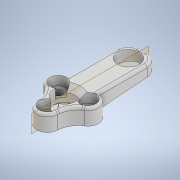
# Autodesk Inventor part: motorholder2
Saved by Autodesk Inventor 2020 (Build 240168000, 168)
## iProperties
Created: 2020-03-28
Part Number: motorholder2
Material: Generic
Document SubType Name: Modeling
Designer: Adam
Density: 1 g/cm^3
Appearance: Default
Author: Adam
Autodesk Inventor part; units mm, degrees
ref_plane "XZ Plane" through (0, 0, 0) normal (0, 1, 0) x (-1, 0, 0)
ref_plane "XY Plane" through (0, 0, 0) normal (0, 0, 1) x (1, 0, 0)
sketch "Sketch2" plane through (0, 0, 0) normal (0, 1, 0) x (-1, 0, 0)
  line L0 (0, 0) -> (10, 0)
  line L1 (10, 0) -> (10, -20)
  line L2 (10, -20) -> (0, -20)
  line L3 (0, -20) -> (0, 0)
  dimension "d0" = 20
  dimension "d1" = 10
  constraints: 8 end point, 2 parallel, 1 horizontal, 1 perpendicular
  measures "d0" distance of L0.end L1.end
  measures "d1" distance of L1.end L2.end
extrude "Extrusion1" add sketch "Sketch2" along normal blind 3
sketch "Sketch3" plane through (0, 3, 0) normal (0, 1, 0) x (1, 0, 0)
  line L0 (-10, 20) -> (-10, 0) projected
  line L1 (0, 20) -> (-10, 20) projected
  line L2 (-10, 0) -> (0, 0) projected
  circle A0 centre (-5, 2.25) radius 0.8
  circle A1 centre (-5, 2.25) radius 1.5
  circle A2 centre (-5, 5.43) radius 2
  point P0 (-4.278066, 3.564843)
  point P1 (-5.721934, 3.564843)
  dimension "d4" = 5
  dimension "d7" = 0
  dimension "d8" = 3.18
  dimension "d10" = 1.6
  dimension "d11" = 2.25
  dimension "d12" = 3
  dimension "d13" = 4
  constraints: 3 centre point, 3 coincident
  measures "d4" distance from line of L0 point (-5, 5.43)
  measures "d7" horizontal distance of point (-5, 5.43) point (-5, 2.25)
  measures "d8" distance of point (-5, 5.43) point (-5, 2.25)
  measures "d10" diameter of A0
  measures "d11" distance from line of L2 A0.centre
  measures "d12" diameter of A1
  measures "d13" diameter of A2
extrude "Extrusion2" cut sketch "Sketch3" against normal through all contours A0
pattern_circular "Circular Pattern1" count 3 over 360 about axis through (-5, 3, -5.43) along (0, 1, 0) of "Extrusion2"
ref_plane "Work Plane2" through (0, 1.3, 0) normal (0, -1, 0) x (1, 0, 0)
ref_plane "Work Plane1" through (0, 0, 0) normal (0, -1, 0) x (1, 0, 0)
extrude "Extrusion3" cut sketch "Sketch3" against normal up to surface (1.7 mm away) contours A0 | A1 A2 | A2 A1 picked at (-5.473989, 3.306122) picked at (-4.949872, 3.544237)
extrude "Extrusion4" cut sketch "Sketch3" against normal through all contours A2 A1 | A1 A2 picked at (-4.949872, 3.544237) picked at (-4.946615, 6.191119)
pattern_circular "Circular Pattern2" count 3 over 360 about axis through (-5, 3, -5.43) along (0, 1, 0) of "Extrusion4", "Extrusion3"
sketch "Sketch6" plane through (0, 3, 0) normal (0, 1, 0) x (1, 0, 0)
  arc A0 (-6.254307, 6.987792) -> (-6.97624, 5.737366) centre (-7.753961, 7.02) ccw
  circle A1 centre (-7.753961, 7.02) radius 1.925
  arc A2 (-3.745693, 6.987792) -> (-6.254307, 6.987792) centre (-5, 5.43) ccw
  circle A3 centre (-5, 2.25) radius 1.925
  circle A4 centre (-2.246039, 7.02) radius 1.925
  arc A5 (-6.923446, 2.172663) -> (-8.78266, 5.392916) centre (-10.920216, 2.011961) ccw
  arc A6 (-1.21734, 5.392916) -> (-3.076554, 2.172663) centre (0.920216, 2.011961) ccw
  arc A7 (-6.859214, 8.724422) -> (-3.140786, 8.724422) centre (-5, 12.266077) ccw
  line L0 (-7.753961, 8.945) -> (-7.753961, 22.712263)
  line L1 (-7.753961, 22.712263) -> (-16.279981, 22.712263)
  line L2 (-16.279981, 22.712263) -> (-16.279981, -9.843768)
  line L3 (-16.279981, -9.843768) -> (12.206544, -9.843768)
  line L4 (12.206544, -9.843768) -> (12.206544, 22.712263)
  line L5 (12.206544, 22.712263) -> (-2.592848, 22.712263)
  line L6 (-2.246039, 8.945) -> (-2.246039, 22.712263)
  point P0 (0, 0)
  point P1 (-1.21734, 5.392916)
  point P2 (-3.076554, 2.172663)
  dimension "d35" = 0.425
  dimension "d38" = 360
  dimension "d40" = 4
  dimension "d43" = 360
  constraints: 14 end point, 8 point on circle, 4 centre point, 4 perpendicular, 3 point on line, 2 vertical, 1 coincident, 1 tangent, 27 other
  measures "d35" radial gap between concentric circles of A1 A0
  measures "d40" radius of A5
extrude "Extrusion5" cut sketch "Sketch6" against normal through all contours A1 A5 A3 A6 A4 L6 L5 L4 L3 L2 L1 L0
fillet "Fillet1" radius 0.5 5 edges at (-5, 3, -0.325) (-2.5439, 3, -4.012) (-0.397, 3, -7.5555) (-9.603, 3, -7.5555) (-7.4561, 3, -4.012)
sketch "Sketch7" plane through (0, 3, 0) normal (0, 1, 0) x (1, 0, 0)
  point P0 (0, 0)
  point P1 (-5.030866, 17.338478)
hole "Hole1" at (-5.030866, 3, -17.338478) direction (0, -1, 0) diameter 4 end through all
fillet "Fillet2" radius 2 2 edges at (-2.246, 1.5, -20) (-7.754, 1.5, -20)
chamfer "Chamfer1" distance 1 angle 45 1 edges at (-5, 3, -7.43)
chamfer "Chamfer2" distance 0.5 angle 45 1 edges at (-4.2781, 0, -7.2952)
ref_plane "Work Plane3" through (-5, 0, -1.45) normal (1, 0, 0) x (0, 1, 0)
sketch "Sketch8" plane through (-5, 0, -1.45) normal (1, 0, 0) x (0, 1, 0)
  line L0 (2.5, -7.495) -> (0, -7.495)
  line L1 (0, -18.55) -> (3, -18.55)
  line L2 (0, -16.55) -> (0, -7.495)
  line L3 (0, -7.495) -> (0.749624, -8.175986) construction
  line L4 (0.749624, -8.175986) -> (0.749624, -18.225203) construction
  line L5 (0.749624, -18.225203) -> (1.5, -18.55) construction
  spline S0 degree 3 poles (0, -7.495) (0.749624, -8.175986) (0.749624, -18.225203) (1.5, -18.55) knots 1 1 1 1 2 2 2 2
  line L6 (0, -7.495) -> (-3.651669, -24.480284)
  line L7 (-3.651669, -24.480284) -> (1.5, -18.55)
  point P0 (0, 1.45)
  constraints: 4 end point, 1 midpoint, 1 parallel, 3 other
extrude "Extrusion6" cut sketch "Sketch8" along normal mid plane 10
fillet "Fillet3" radius 2 2 edges at (-3.623, 0, -8.945) (-6.377, 0, -8.945)
fillet "Fillet4" radius 0.5 5 edges at (-7.1682, 3, -19.4142) (-5, 3, -20) (-2.8318, 3, -19.4142) (-2.246, 3, -13.26) (-7.754, 3, -13.26)
equation "\"d4\" = 0.5 * d1"
body "Solid1"
